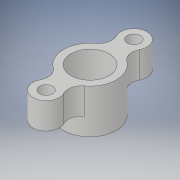
# Autodesk Inventor part: Cap
Saved by Autodesk Inventor 2019 (Build 230136000, 136)
## iProperties
Created: 2019-10-09
Part Number: Cap
Material: Generic
Document SubType Name: Modeling
Designer: 19879326
Density: 1 g/cm^3
Appearance: Default
Author: 19879326
Autodesk Inventor part; units mm, degrees
ref_plane "YZ Plane" through (0, 0, 0) normal (1, 0, 0) x (0, 1, 0)
ref_plane "XZ Plane" through (0, 0, 0) normal (0, 1, 0) x (-1, 0, 0)
ref_plane "XY Plane" through (0, 0, 0) normal (0, 0, 1) x (1, 0, 0)
sketch "Sketch1" plane through (0, 0, 0) normal (0, 1, 0) x (-1, 0, 0)
  circle A0 centre (0, 10) radius 1.5
  circle A1 centre (0, -10) radius 1.5
  arc A2 (2.6663, 8.625) -> (-2.6663, 8.625) centre (0, 10) ccw
  arc A3 (-2.6663, -8.625) -> (2.6663, -8.625) centre (0, -10) ccw
  arc A4 (2.6663, 8.625) -> (3.5551, 4.8333) centre (5.3327, 7.25) ccw
  arc A5 (-3.5551, 4.8333) -> (-2.6663, 8.625) centre (-5.3327, 7.25) ccw
  arc A6 (3.5551, -4.8333) -> (2.6663, -8.625) centre (5.3327, -7.25) ccw
  arc A7 (-2.6663, -8.625) -> (-3.5551, -4.8333) centre (-5.3327, -7.25) ccw
  arc A8 (-3.5551, 4.8333) -> (-3.5551, -4.8333) centre (0, 0) ccw
  arc A9 (3.5551, -4.8333) -> (3.5551, 4.8333) centre (0, 0) ccw
  dimension "d1" = 10
  dimension "d2" = 20
  dimension "d3" = 3
  dimension "d4" = 6
  dimension "d5" = 6
  dimension "d6" = 6
  dimension "d7" = 6
  dimension "d8" = 3
  constraints: 16 point on circle, 10 centre point, 5 tangent, 4 equal radius, 4 vertical alignment, 3 coincident, 2 horizontal alignment
  measures "d1" distance of point (0, 0) A0.centre
  measures "d2" distance of A1.centre A0.centre
  measures "d3" diameter of A0
  measures "d4" diameter of A2
  measures "d5" diameter of A3
  measures "d6" radius of A9
  measures "d7" radius of A8
  measures "d8" radius of A5
extrude "Extrusion1" add sketch "Sketch1" along normal blind 10
sketch "Sketch2" plane through (0, 10, 0) normal (0, 1, 0) x (1, 0, 0)
  circle A0 centre (0, 0) radius 4.35
  dimension "d11" = 8.7
  constraints: 1 centre point, 1 coincident
  measures "d11" diameter of A0
extrude "Extrusion2" cut sketch "Sketch2" against normal blind 8
sketch "Sketch3" plane through (0, 0, 0) normal (0, -1, 0) x (1, 0, 0)
  circle A0 centre (0, 10) radius 1.5 projected
  arc A1 (2.6663, 8.625) -> (-2.6663, 8.625) centre (0, 10) ccw
  circle A2 centre (0, -10) radius 1.5 projected
  arc A3 (-2.6663, -8.625) -> (2.6663, -8.625) centre (0, -10) ccw
  arc A4 (2.6663, 8.625) -> (-2.6663, 8.625) centre (0, 10) ccw projected
  arc A5 (2.6663, 8.625) -> (3.5551, 4.8333) centre (5.3327, 7.25) ccw
  arc A6 (-3.5551, 4.8333) -> (-2.6663, 8.625) centre (-5.3327, 7.25) ccw
  arc A7 (-2.6663, -8.625) -> (-3.5551, -4.8333) centre (-5.3327, -7.25) ccw
  arc A8 (3.5551, -4.8333) -> (2.6663, -8.625) centre (5.3327, -7.25) ccw
  arc A9 (3.5551, -4.8333) -> (3.5551, 4.8333) centre (0, 0) ccw projected
  arc A10 (2.6663, 8.625) -> (3.5551, 4.8333) centre (5.3327, 7.25) ccw projected
  arc A11 (-3.5551, 4.8333) -> (-2.6663, 8.625) centre (-5.3327, 7.25) ccw projected
  arc A12 (-2.6663, -8.625) -> (-3.5551, -4.8333) centre (-5.3327, -7.25) ccw projected
  arc A13 (3.5551, -4.8333) -> (2.6663, -8.625) centre (5.3327, -7.25) ccw projected
  arc A14 (-3.5551, 4.8333) -> (-3.5551, -4.8333) centre (0, 0) ccw projected
  arc A15 (-2.6663, -8.625) -> (2.6663, -8.625) centre (0, -10) ccw projected
  arc A16 (3.5551, 4.8333) -> (-3.5551, 4.8333) centre (0, 0) ccw
  arc A17 (-3.5551, -4.8333) -> (3.5551, -4.8333) centre (0, 0) ccw
  constraints: 29 point on circle, 11 tangent, 8 centre point, 3 coincident, 2 equal radius
extrude "Extrusion3" cut sketch "Sketch3" against normal blind 4 contours A5 A16 A6 A1 | A8 A3 A7 A17
body "Solid1"
